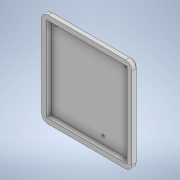
# Autodesk Inventor part: Tampa
Saved by Autodesk Inventor 2021 (Build 250183000, 183)
## iProperties
Created: 2020-12-21
Part Number: Tampa
Material: Generic
Document SubType Name: Modeling
Designer: Vitor
Density: 1 g/cm^3
Appearance: Default
Author: Vitor
Autodesk Inventor part; units mm, degrees
ref_plane "YZ Plane" through (0, 0, 0) normal (1, 0, 0) x (0, 1, 0)
ref_plane "XZ Plane" through (0, 0, 0) normal (0, 1, 0) x (-1, 0, 0)
ref_plane "XY Plane" through (0, 0, 0) normal (0, 0, 1) x (1, 0, 0)
sketch "Sketch1" plane through (0, 0, 0) normal (0, 0, 1) x (1, 0, 0)
  line L0 (0, 103.81) -> (0, 0)
  line L1 (99.04, 103.81) -> (0, 103.81)
  line L2 (99.04, 0) -> (99.04, 103.81)
  circle A0 centre (91.5302, 97.8155) radius 1.6
  circle A1 centre (6.3166, 98.2023) radius 1.6
  circle A2 centre (63.7434, 9.4559) radius 1.6
  line L3 (-2.8877, 39.67) -> (-2.8877, 25.07)
  line L4 (18.04, 39.67) -> (-2.8877, 39.67)
  line L5 (-2.8877, 25.07) -> (18.04, 25.07)
  line L6 (5.99, 20.97) -> (-0.5, 20.97)
  line L7 (-0.5, 20.97) -> (-0.5, 9.286)
  line L8 (-0.5, 9.286) -> (5.99, 9.286)
  line L9 (5.99, 9.286) -> (5.99, 20.97)
  line L10 (18.04, 25.07) -> (18.04, 39.67)
  line L11 (0, 0) -> (99.04, 0)
  line L12 (-2, 105.81) -> (-2, -2)
  line L13 (-2, -2) -> (101.04, -2)
  line L14 (101.04, -2) -> (101.04, 105.81)
  line L15 (101.04, 105.81) -> (-2, 105.81)
  line L16 (-6, 109.81) -> (-6, -6)
  line L17 (-6, -6) -> (105.04, -6)
  line L18 (105.04, -6) -> (105.04, 109.81)
  line L19 (105.04, 109.81) -> (-6, 109.81)
  point P0 (0, 20.97)
  point P1 (0, 9.286)
  dimension "d0" = 2
  dimension "d1" = 4
  constraints: 40 end point, 3 centre point, 2 horizontal, 2 vertical, 6 other
  measures "d0" distance between parallel lines of L1 L15
  measures "d1" distance between parallel lines of L15 L19
extrude "Extrusion1" add sketch "Sketch1" along normal blind 8 contours L0 L4 L12 L15 L14 L13 L5 L6 L7 L8 L11 L2 L1 | L0 L5 L12 L4 | L12 L5 L3 L4 | L0 L8 L7 L6 | L19 L18 L17 L16
extrude "Extrusion2" add sketch "Sketch1" along normal blind 2 contours L1 L2 L11 L0 L8 L9 L6 L5 L10 L4 | L4 L10 L5 L0 | L6 L9 L8 L0 | L0 L8 L7 L6
fillet "Fillet1" radius 8 4 edges at (-6, -6, 4) (-6, 109.81, 4) (105.04, 109.81, 4) (105.04, -6, 4)
chamfer "Chamfer1" distance 3 angle 45 8 edges at (-6, 51.905, 0) (-3.6569, -3.6569, 0) (49.52, -6, 0) (102.6969, -3.6569, 0) (105.04, 51.905, 0) (102.6969, 107.4669, 0) (49.52, 109.81, 0) (-3.6569, 107.4669, 0)
body "Solid1"
